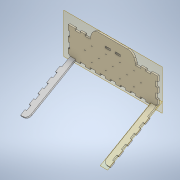
# Autodesk Inventor part: mounting_points
Saved by Autodesk Inventor 2020 (Build 240168000, 168)
## iProperties
Created: 2019-08-02
Part Number: mounting_points
Material: Generic
Document SubType Name: Modeling
Designer: erwin
Density: 1 g/cm^3
Appearance: Default
Author: erwin
Autodesk Inventor part; units mm, degrees
ref_plane "YZ Plane" through (0, 0, 0) normal (1, 0, 0) x (0, 1, 0)
ref_plane "XZ Plane" through (0, 0, 0) normal (0, 1, 0) x (-1, 0, 0)
ref_plane "XY Plane" through (0, 0, 0) normal (0, 0, 1) x (1, 0, 0)
ref_plane "Work Plane1" through (0, 0, 0) normal (0, 0, 1) x (1, 0, 0)
sketch "Sketch1" plane through (0, 0, 0) normal (0, 0, 1) x (1, 0, 0)
  line L0 (54, 88) -> (54, 100) projected
  line L1 (18, 88) -> (54, 88) projected
  line L2 (18, 100) -> (18, 88) projected
  line L3 (18, 100) -> (54, 100) projected
  line L4 (-18, 88) -> (-18, 100) projected
  line L5 (-54, 88) -> (-18, 88) projected
  line L6 (-54, 100) -> (-54, 88) projected
  line L7 (-54, 100) -> (-18, 100) projected
  line L8 (162, 100) -> (150.6253, 128.5218) projected
  arc A0 (150.6253, 128.5218) -> (104.1824, 160) centre (104.1824, 110) ccw projected
  line L9 (104.1824, 160) -> (-104.1824, 160) projected
  arc A1 (-104.1824, 160) -> (-150.6253, 128.5218) centre (-104.1824, 110) ccw projected
  line L10 (-150.6253, 128.5218) -> (-162, 100) projected
  line L11 (-162, 88) -> (-162, 100) projected
  line L12 (-198, 88) -> (-162, 88) projected
  line L13 (-198, 100) -> (-198, 88) projected
  line L14 (-234, 100) -> (-198, 100) projected
  line L15 (-234, 88) -> (-234, 100) projected
  line L16 (-270, 88) -> (-234, 88) projected
  line L17 (-270, 100) -> (-270, 88) projected
  line L18 (-318, 100) -> (-270, 100) projected
  line L19 (-318, 64) -> (-318, 100) projected
  line L20 (-306, 64) -> (-318, 64) projected
  line L21 (-306, 28) -> (-306, 64) projected
  line L22 (-318, 28) -> (-306, 28) projected
  line L23 (-318, -8) -> (-318, 28) projected
  line L24 (-306, -8) -> (-318, -8) projected
  line L25 (-306, -44) -> (-306, -8) projected
  line L26 (-318, -44) -> (-306, -44) projected
  line L27 (-318, -80) -> (-318, -44) projected
  line L28 (-306, -80) -> (-318, -80) projected
  line L29 (-306, -88) -> (-306, -80) projected
  line L30 (-270, -88) -> (-306, -88) projected
  line L31 (-270, -100) -> (-270, -88) projected
  line L32 (-234, -100) -> (-270, -100) projected
  line L33 (-234, -88) -> (-234, -100) projected
  line L34 (-198, -88) -> (-234, -88) projected
  line L35 (-198, -100) -> (-198, -88) projected
  line L36 (-162, -100) -> (-198, -100) projected
  line L37 (-162, -88) -> (-162, -100) projected
  line L38 (-126, -88) -> (-162, -88) projected
  line L39 (-126, -100) -> (-126, -88) projected
  line L40 (-90, -100) -> (-126, -100) projected
  line L41 (-90, -88) -> (-90, -100) projected
  line L42 (-54, -88) -> (-90, -88) projected
  line L43 (-54, -100) -> (-54, -88) projected
  line L44 (-18, -100) -> (-54, -100) projected
  line L45 (-18, -88) -> (-18, -100) projected
  line L46 (18, -88) -> (-18, -88) projected
  line L47 (18, -100) -> (18, -88) projected
  line L48 (54, -100) -> (18, -100) projected
  line L49 (54, -88) -> (54, -100) projected
  line L50 (90, -88) -> (54, -88) projected
  line L51 (90, -100) -> (90, -88) projected
  line L52 (126, -100) -> (90, -100) projected
  line L53 (126, -88) -> (126, -100) projected
  line L54 (162, -88) -> (126, -88) projected
  line L55 (162, -100) -> (162, -88) projected
  line L56 (198, -100) -> (162, -100) projected
  line L57 (198, -88) -> (198, -100) projected
  line L58 (234, -88) -> (198, -88) projected
  line L59 (234, -100) -> (234, -88) projected
  line L60 (270, -100) -> (234, -100) projected
  line L61 (270, -88) -> (270, -100) projected
  line L62 (306, -88) -> (270, -88) projected
  line L63 (306, -80) -> (306, -88) projected
  line L64 (318, -80) -> (306, -80) projected
  line L65 (318, -44) -> (318, -80) projected
  line L66 (306, -44) -> (318, -44) projected
  line L67 (306, -8) -> (306, -44) projected
  line L68 (318, -8) -> (306, -8) projected
  line L69 (318, 28) -> (318, -8) projected
  line L70 (306, 28) -> (318, 28) projected
  line L71 (306, 64) -> (306, 28) projected
  line L72 (318, 64) -> (306, 64) projected
  line L73 (318, 100) -> (318, 64) projected
  line L74 (270, 100) -> (318, 100) projected
  line L75 (270, 88) -> (270, 100) projected
  line L76 (234, 88) -> (270, 88) projected
  line L77 (234, 100) -> (234, 88) projected
  line L78 (198, 100) -> (234, 100) projected
  line L79 (198, 88) -> (198, 100) projected
  line L80 (162, 88) -> (198, 88) projected
  line L81 (162, 100) -> (162, 88) projected
  circle A2 centre (-50, -50) radius 2.5 projected
  circle A3 centre (150, -50) radius 2.5 projected
  circle A4 centre (-150, 50) radius 2.5 projected
  circle A5 centre (50, 50) radius 2.5 projected
  circle A6 centre (150, 50) radius 2.5 projected
  circle A7 centre (-100, 0) radius 2.5 projected
  circle A8 centre (-200, 0) radius 2.5 projected
  circle A9 centre (200, 0) radius 2.5 projected
  circle A10 centre (100, 0) radius 2.5 projected
  circle A11 centre (0, 0) radius 2.5 projected
  circle A12 centre (-50, 50) radius 2.5 projected
  circle A13 centre (50, -50) radius 2.5 projected
  circle A14 centre (-150, -50) radius 2.5 projected
  point P0 (0, 0)
ref_plane "Work Plane2" through (294, -186.3946, 163.1655) normal (0, 0.866, 0.5) x (1, 0, 0)
sketch "Sketch2" plane through (294, -186.3946, 163.1655) normal (0, 0.866, 0.5) x (1, 0, 0)
  line L0 (24, -205) -> (6, -205) projected
  line L1 (24, -168.25) -> (24, -205) projected
  line L2 (12, -168.25) -> (24, -168.25) projected
  line L3 (12, -133.75) -> (12, -168.25) projected
  line L4 (24, -133.75) -> (12, -133.75) projected
  line L5 (24, -96.25) -> (24, -133.75) projected
  line L6 (12, -96.25) -> (24, -96.25) projected
  line L7 (12, -61.75) -> (12, -96.25) projected
  line L8 (24, -61.75) -> (12, -61.75) projected
  line L9 (24, -24.25) -> (24, -61.75) projected
  line L10 (12, -24.25) -> (24, -24.25) projected
  line L11 (12, 10.25) -> (12, -24.25) projected
  line L12 (24, 10.25) -> (12, 10.25) projected
  line L13 (24, 47.75) -> (24, 10.25) projected
  line L14 (12, 47.75) -> (24, 47.75) projected
  line L15 (12, 82.25) -> (12, 47.75) projected
  line L16 (24, 82.25) -> (12, 82.25) projected
  line L17 (24, 119.75) -> (24, 82.25) projected
  line L18 (12, 119.75) -> (24, 119.75) projected
  line L19 (12, 205) -> (12, 119.75) projected
  line L20 (-24, 205) -> (12, 205) projected
  line L21 (-24, -175) -> (-24, 205) projected
  arc A0 (-24, -175) -> (6, -205) centre (6, -175) ccw projected
  line L22 (-612, -204.25) -> (-594, -204.25) projected
  arc A1 (-594, -204.25) -> (-564, -174.25) centre (-594, -174.25) ccw projected
  line L23 (-564, -174.25) -> (-564, 205.75) projected
  line L24 (-564, 205.75) -> (-600, 205.75) projected
  line L25 (-600, 205.75) -> (-600, 120.5) projected
  line L26 (-600, 120.5) -> (-612, 120.5) projected
  line L27 (-612, 120.5) -> (-612, 83) projected
  line L28 (-612, 83) -> (-600, 83) projected
  line L29 (-600, 83) -> (-600, 48.5) projected
  line L30 (-600, 48.5) -> (-612, 48.5) projected
  line L31 (-612, 48.5) -> (-612, 11) projected
  line L32 (-612, 11) -> (-600, 11) projected
  line L33 (-600, 11) -> (-600, -23.5) projected
  line L34 (-600, -23.5) -> (-612, -23.5) projected
  line L35 (-612, -23.5) -> (-612, -61) projected
  line L36 (-612, -61) -> (-600, -61) projected
  line L37 (-600, -61) -> (-600, -95.5) projected
  line L38 (-600, -95.5) -> (-612, -95.5) projected
  line L39 (-612, -95.5) -> (-612, -133) projected
  line L40 (-612, -133) -> (-600, -133) projected
  line L41 (-600, -133) -> (-600, -167.5) projected
  line L42 (-600, -167.5) -> (-612, -167.5) projected
  line L43 (-612, -167.5) -> (-612, -204.25) projected
  point P0 (-294, 234.5028)
extrude "Extrusion1" add sketch "Sketch1" against normal blind 12
extrude "Extrusion2" add sketch "Sketch2" against normal blind 12
body "Solid1"
